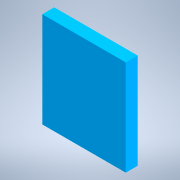
# Autodesk Inventor part: ToF Sensor6
Saved by Autodesk Inventor 2022.3 (Build 263350000, 350)
## iProperties
Created: 2023-02-07
Part Number: ToF Sensor6
Material: Generic
Document SubType Name: Modeling
Designer: lbmcgill42
Density: 1 g/cm^3
Appearance: Default
Author: lbmcgill42
Autodesk Inventor part; units mm, degrees
ref_plane "YZ Plane" through (0, 0, 0) normal (1, 0, 0) x (0, 1, 0)
ref_plane "XZ Plane" through (0, 0, 0) normal (0, 1, 0) x (-1, 0, 0)
ref_plane "XY Plane" through (0, 0, 0) normal (0, 0, 1) x (1, 0, 0)
sketch "Sketch1" plane through (0, 0, 0) normal (0, 0, 1) x (1, 0, 0)
  line L0 (-6.8025, 3.7935) -> (10.9775, 3.7935)
  line L1 (10.9775, 3.7935) -> (10.9775, -16.5265)
  line L2 (10.9775, -16.5265) -> (-6.8025, -16.5265)
  line L3 (-6.8025, -16.5265) -> (-6.8025, 3.7935)
  point P0 (0, 0)
  dimension "d0" = 17.78
  dimension "d1" = 20.32
  constraints: 8 end point, 2 parallel, 1 horizontal, 1 perpendicular
  measures "d0" distance of L1.end L2.end
  measures "d1" distance of L0.end L1.end
extrude "Extrusion1" add sketch "Sketch1" along normal blind 2.54
body "Solid1"
